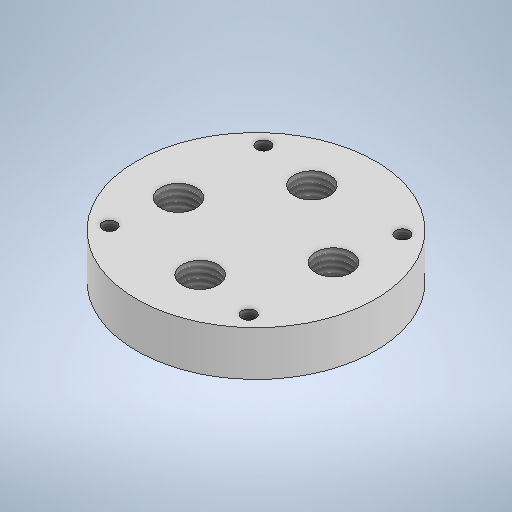
# Autodesk Inventor part: Part7
Saved by Autodesk Inventor 2025 (Build 290162000, 162)
## iProperties
Created: 2026-06-20
Part Number: Part7
Material: Generic
Document SubType Name: Modeling
Designer: saket
Density: 1 g/cm^3
Appearance: Default
Author: saket
Autodesk Inventor part; units mm, degrees
ref_plane "YZ Plane" through (0, 0, 0) normal (1, 0, 0) x (0, 1, 0)
ref_plane "XZ Plane" through (0, 0, 0) normal (0, 1, 0) x (-1, 0, 0)
ref_plane "XY Plane" through (0, 0, 0) normal (0, 0, 1) x (1, 0, 0)
sketch "Sketch1" plane through (0, 0, 0) normal (0, 1, 0) x (-1, 0, 0)
  circle A0 centre (0, 0) radius 26.67
  circle A1 centre (2.413, -14.8844) radius 0.6
  circle A2 centre (2.413, -14.8844) radius 4.0005
  circle A3 centre (14.8844, 2.413) radius 4.0005
  circle A4 centre (14.8844, 2.413) radius 0.6
  circle A5 centre (-2.413, 14.8844) radius 4.0005
  circle A6 centre (-2.413, 14.8844) radius 0.6
  circle A7 centre (-14.8844, -2.413) radius 4.0005
  circle A8 centre (-14.8844, -2.413) radius 0.6
  circle A9 centre (15.5194, -17.1704) radius 1.524
  circle A10 centre (17.1704, 15.5194) radius 1.524
  circle A11 centre (-15.5194, 17.1704) radius 1.524
  circle A12 centre (-17.1704, -15.5194) radius 1.524
  dimension "d0" = 53.34
  dimension "d7" = 360
  dimension "d14" = 360
  constraints: 13 centre point, 5 coincident, 26 other
  measures "d0" diameter of A0
extrude "Extrusion1" add sketch "Sketch1" against normal blind 10.0076 contours A0 | A2 | A3 | A5 | A7 | A8
hole "Hole1" at (-14.8844, 0, 2.413) direction (0, -1, 0) diameter 8 depth 7.493
hole "Hole2" at (-2.413, 0, -14.8844) at (2.413, 0, 14.8844) at (14.8844, 0, -2.413) direction (0, -1, 0) diameter 8 depth 7.493
hole "Hole3" at (14.8844, 0, -2.413) direction (0, -1, 0) diameter 1.2 end through all
thread "Thread1" size "M3x0.5" class "6H" standard "ANSI Metric M Profile" length 10
thread "Thread2" size "M3x0.5" class "6H" standard "ANSI Metric M Profile" length 10
thread "Thread3" size "M3x0.5" class "6H" standard "ANSI Metric M Profile" length 10
thread "Thread4" size "M3x0.5" class "6H" standard "ANSI Metric M Profile" length 10
thread "Thread5" size "M8x1.25" class "6H" standard "ANSI Metric M Profile" length 10
thread "Thread6" size "M8x1.25" class "6H" standard "ANSI Metric M Profile" length 10
thread "Thread7" size "M8x1.25" class "6H" standard "ANSI Metric M Profile" length 10
thread "Thread8" size "M8x1.25" class "6H" standard "ANSI Metric M Profile" length 10
body "Solid1"
